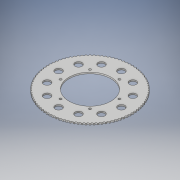
# Autodesk Inventor part: Corona92T
Saved by Autodesk Inventor 2018 (Build 220112000, 112)
## iProperties
Created: 2017-11-17
Part Number: Corona92T
Material: Generic
Document SubType Name: Modeling
Designer: eroldan
Density: 1 g/cm^3
Appearance: Default
Author: eroldan
Autodesk Inventor part; units mm, degrees
ref_plane "YZ Plane" through (0, 0, 0) normal (1, 0, 0) x (0, 1, 0)
ref_plane "XZ Plane" through (0, 0, 0) normal (0, 1, 0) x (-1, 0, 0)
ref_plane "XY Plane" through (0, 0, 0) normal (0, 0, 1) x (1, 0, 0)
sketch "Sketch1" plane through (0, 0, 0) normal (0, 0, 1) x (1, 0, 0)
  circle A0 centre (0, 0) radius 116.5
  dimension "d0" = 233
  constraints: 1 centre point, 1 coincident
  measures "d0" diameter of A0
extrude "Extrusion1" add sketch "Sketch1" along normal mid plane 4
sketch "Sketch2" plane through (0, 0, 2) normal (0, 0, 1) x (1, 0, 0)
  circle A0 centre (0, 87) radius 9.5
  circle A1 centre (-43.5, 75.3442) radius 9.5
  circle A2 centre (-75.3442, 43.5) radius 9.5
  circle A3 centre (-87, 0) radius 9.5
  circle A4 centre (-75.3442, -43.5) radius 9.5
  circle A5 centre (-43.5, -75.3442) radius 9.5
  circle A6 centre (0, -87) radius 9.5
  circle A7 centre (43.5, -75.3442) radius 9.5
  circle A8 centre (75.3442, -43.5) radius 9.5
  circle A9 centre (87, 0) radius 9.5
  circle A10 centre (75.3442, 43.5) radius 9.5
  circle A11 centre (43.5, 75.3442) radius 9.5
  circle A12 centre (0, 0) radius 58
  line L0 (-75.3442, 43.5) -> (-43.5, 75.3442) construction
  line L1 (-59.4221, 59.4221) -> (0, 0) construction
  point P0 (-47.1463, 47.1463)
  dimension "d3" = 19
  dimension "d6" = 360
  dimension "d11" = 116
  dimension "d25" = 66.675
  dimension "d36" = 87
  constraints: 13 centre point, 4 end point, 1 coincident, 1 midpoint, 25 other
  measures "d3" diameter of A0
  measures "d11" diameter of A12
  measures "d25" distance of point (0, 0) point (-47.146, 47.146)
  measures "d36" distance of point (0, 0) A0.centre
extrude "Extrusion2" cut sketch "Sketch2" against normal blind 116
sketch "Sketch4" plane through (0, 0, 2) normal (0, 0, 1) x (1, 0, 0)
  point P0 (0, 0)
  point P1 (0, 116.4955)
hole "Hole1" at (0, 116.4955, 2) direction (0, 0, -1) diameter 5 end through all
pattern_circular "Circular Pattern1" count 92 over 360 about axis through (0, 0, -10) along (0, 0, 1) of "Hole1"
hole "Hole2" at (-47.1463, 47.1463, 2) direction (0, 0, -1) diameter 6.35 end through all
pattern_circular "Circular Pattern2" count 6 over 360 about axis through (0, 0, -10) along (0, 0, 1) of "Hole2"
equation "\"d8\" = d11"
body "Solid1"
